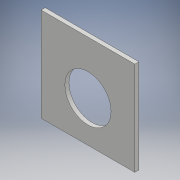
# Autodesk Inventor part: field-mover-motor-case
Saved by Autodesk Inventor 2017 (Build 210142000, 142)
## iProperties
Created: 2017-03-05
Part Number: field-mover-motor-case
Material: Generic
Document SubType Name: Modeling
Designer: John
Density: 1 g/cm^3
Appearance: Default
Author: John
Autodesk Inventor part; units mm, degrees
ref_plane "YZ Plane" through (0, 0, 0) normal (1, 0, 0) x (0, 1, 0)
ref_plane "XZ Plane" through (0, 0, 0) normal (0, 1, 0) x (-1, 0, 0)
ref_plane "XY Plane" through (0, 0, 0) normal (0, 0, 1) x (1, 0, 0)
sketch "Sketch1" plane through (0, 0, 0) normal (0, 1, 0) x (-1, 0, 0)
  line L0 (0, 0) -> (-69, 0)
  line L1 (-69, 0) -> (-69, 69)
  line L2 (-69, 69) -> (0, 69)
  line L3 (0, 69) -> (0, 0)
  circle A0 centre (-34.5, 30) radius 17
  line L4 (-34.5, 30) -> (-69, 30) construction
  line L5 (-34.5, 30) -> (0, 30) construction
  dimension "d0" = 69
  dimension "d1" = 69
  dimension "d2" = 34
  dimension "d5" = 30
  constraints: 12 end point, 3 point on line, 2 parallel, 2 perpendicular, 1 centre point, 1 collinear, 1 horizontal
  measures "d0" distance of L1.end L2.end
  measures "d1" distance of L0.end L1.end
  measures "d2" diameter of A0
  measures "d5" distance from line of L0 L4.start
extrude "Extrusion1" add sketch "Sketch1" along normal blind 3
body "Solid1"
